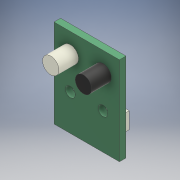
# Autodesk Inventor part: IR모듈
Saved by Autodesk Inventor 2017 (Build 210142000, 142)
## iProperties
Part Number: IR모듈
Material: 일반
Document SubType Name: Modeling
Designer: minom
Density: 1 g/cm^3
Appearance: 기본값
Mass: 1.58735 g
Surface Area: 16.4592 cm^2
Volume: 1.58735 cm^3
Author: minom
Autodesk Inventor part; units mm, degrees
ref_plane "YZ Plane" through (0, 0, 0) normal (1, 0, 0) x (0, 1, 0)
ref_plane "XZ Plane" through (0, 0, 0) normal (0, 1, 0) x (-1, 0, 0)
ref_plane "XY Plane" through (0, 0, 0) normal (0, 0, 1) x (1, 0, 0)
sketch "스케치1" plane through (0, 0, 0) normal (0, 1, 0) x (-1, 0, 0)
  line L0 (0, 0) -> (-20, 0)
  line L1 (-20, 0) -> (-20, 27)
  line L2 (-20, 27) -> (0, 27)
  line L3 (0, 27) -> (0, 0)
  dimension "d0" = 20
  dimension "d1" = 27
  constraints: 8 end point, 2 parallel, 1 horizontal, 1 perpendicular
  measures "d0" distance of L1.end L2.end
  measures "d1" distance of L0.end L1.end
extrude "돌출1" add sketch "스케치1" along normal blind 2
sketch "스케치2" plane through (0, 2, 0) normal (0, 1, 0) x (1, 0, 0)
  line L0 (20, 0) -> (0, 0) projected
  line L1 (0, 0) -> (0, -27) projected
  line L2 (0, -27) -> (20, -27) projected
  line L3 (20, -27) -> (20, 0) projected
  line L4 (20, 0) -> (0, 0) projected
  circle A0 centre (5, -11) radius 1.5
  circle A1 centre (15, -11) radius 1.5
  dimension "d5" = 3
  dimension "d6" = 3
  dimension "d21" = 5
  dimension "d22" = 5
  dimension "d23" = 11
  dimension "d24" = 11
  constraints: 2 centre point
  measures "d5" diameter of A0
  measures "d6" diameter of A1
  measures "d21" distance from line of L3 A1.centre
  measures "d22" distance from line of L1 A0.centre
  measures "d23" distance from line of L0 A0.centre
  measures "d24" distance from line of L0 A1.centre
extrude "돌출2" cut sketch "스케치2" against normal blind 2 contours A0 | A1
sketch "스케치3" plane through (0, 0, 0) normal (0, -1, 0) x (1, 0, 0)
  circle A0 centre (5, 11) radius 1.5 projected
  circle A1 centre (15, 11) radius 1.5 projected
  line L0 (0, 0) -> (20, 0) projected
  line L1 (20, 0) -> (20, 27) projected
  line L2 (20, 27) -> (0, 27) projected
  line L3 (0, 27) -> (0, 0) projected
  line L4 (5, 11) -> (5, 21)
  line L5 (15, 11) -> (15, 21)
  circle A2 centre (5, 21) radius 2.5
  circle A3 centre (15, 21) radius 2.5
  dimension "d9" = 10
  dimension "d10" = 5
  dimension "d11" = 5
  constraints: 4 end point, 2 centre point, 2 coincident, 1 vertical
  measures "d9" distance of L4.start L4.end
  measures "d10" diameter of A2
  measures "d11" diameter of A3
extrude "돌출3" add sketch "스케치3" along normal blind 6 contours A2 | A3
sketch "스케치4" plane through (0, 2, 0) normal (0, 1, 0) x (1, 0, 0)
  circle A0 centre (5, -11) radius 1.5 projected
  circle A1 centre (15, -11) radius 1.5 projected
  line L0 (20, 0) -> (0, 0) projected
  line L1 (0, 0) -> (0, -27) projected
  line L2 (0, -27) -> (20, -27) projected
  line L3 (20, -27) -> (20, 0) projected
  line L4 (0, 0) -> (20, 0) projected
  line L5 (5, -2) -> (15, -2)
  line L6 (15, -2) -> (15, -7)
  line L7 (15, -7) -> (5, -7)
  line L8 (5, -7) -> (5, -2)
  dimension "d14" = 2
  constraints: 8 end point, 2 parallel, 1 horizontal, 1 perpendicular
  measures "d14" distance between parallel lines of L5 L0
extrude "돌출4" add sketch "스케치4" along normal blind 6 contours L5 L6 L7 L8
